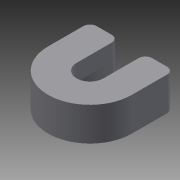
# Autodesk Inventor part: HeadConnector
Saved by Autodesk Inventor 2014 SP1 (Build 180222100, 222)
## iProperties
Created: 2013-10-30
Part Number: HeadConnector
Material: Generic
Document SubType Name: Modeling
Designer: david
Density: 1 g/cm^3
Appearance: Default
HeadConnectorDiam: 20,000 mm
HeadConnectorHeight: 5,000 mm
HeadConnectorOuterSize: 25,000 mm
HeadConnectorWidth: 8,000 mm
HeadConnectorOuterHeight: 5,000 mm
HeadConnectorTolerance: 0,200 mm
Author: david
Autodesk Inventor part; units mm, degrees
ref_plane "YZ Plane" through (0, 0, 0) normal (1, 0, 0) x (0, 1, 0)
ref_plane "XZ Plane" through (0, 0, 0) normal (0, 1, 0) x (-1, 0, 0)
ref_plane "XY Plane" through (0, 0, 0) normal (0, 0, 1) x (1, 0, 0)
sketch "Sketch1" plane through (0, 0, 0) normal (0, 1, 0) x (-1, 0, 0)
  arc A0 (12.5, 0) -> (-12.5, 0) centre (0, 0) ccw
  arc A1 (4, 0) -> (-4, 0) centre (0, 0) ccw
  line L0 (-12.5, 0) -> (12.5, 0) construction
  line L1 (0, 0) -> (0, -12.6122) construction
  line L2 (-12.5, 0) -> (-12.5, -12.5)
  line L3 (-4, 0) -> (-4, -12.5)
  line L4 (4, 0) -> (4, -12.5)
  line L5 (12.5, 0) -> (12.5, -12.5)
  line L6 (-12.5, -12.5) -> (-4, -12.5)
  line L7 (4, -12.5) -> (12.5, -12.5)
  dimension "d0" = 25
  dimension "d2" = 12.5
  dimension "d3" = 8
  dimension "d6" = 12.5
  dimension "d8" = 12.5
  constraints: 16 end point, 4 point on circle, 4 tangent, 3 parallel, 2 centre point, 2 coincident, 2 point on line, 1 horizontal, 1 perpendicular
  measures "d0" distance of L0.end L0.start
  measures "d2" radius of A0
  measures "d3" distance of L3.start L4.start
  measures "d6" distance of L2.end L0.start
  measures "d8" distance from line of L1.end L5
extrude "Extrusion1" add sketch "Sketch1" against normal blind 5
sketch "Sketch2" plane through (0, -5, 0) normal (0, -1, 0) x (1, 0, 0)
  arc A0 (12.5, 0) -> (-12.5, 0) centre (0, 0) ccw projected
  line L0 (-12.5, 0) -> (-12.5, -12.5) projected
  line L1 (-4, -12.5) -> (-4, 0) projected
  arc A1 (4, 0) -> (-4, 0) centre (0, 0) ccw projected
  line L2 (4, 0) -> (4, -12.5) projected
  line L3 (12.5, -12.5) -> (12.5, 0) projected
  arc A2 (4, -9.1652) -> (-4, -9.1652) centre (0, 0) ccw
  arc A3 (12.5, 0) -> (-12.5, 0) centre (0, 0) ccw
  line L4 (-12.5, 0) -> (-12.5, -12.5)
  line L5 (-4, -12.5) -> (-4, -9.1652)
  line L6 (4, -9.1652) -> (4, -12.5)
  line L7 (12.5, -12.5) -> (12.5, 0)
  line L8 (-12.5, -12.5) -> (-4, -12.5)
  line L9 (4, -12.5) -> (12.5, -12.5)
  dimension "d11" = 10
  constraints: 12 end point, 5 point on circle, 4 tangent, 3 collinear, 2 centre point, 2 coincident, 2 point on line, 1 parallel, 1 perpendicular
  measures "d11" radius of A2
extrude "Extrusion2" add sketch "Sketch2" along normal blind 5 contours L3 L9 L2 A2 L1 L8 L0 A0
fillet "Fillet1" radius 2 1 edges at (12.5, -5, -12.5)
fillet "Fillet2" radius 2 3 edges at (4, -5, -12.5) (-4, -5, -12.5) (-12.5, -5, -12.5)
sketch "Sketch3" plane through (0, -5, 0) normal (0, -1, 0) x (1, 0, 0)
  arc A0 (4, -9.1652) -> (-4, -9.1652) centre (0, 0) ccw projected
  line L0 (-4, -9.1652) -> (-4, 0) projected
  arc A1 (4, 0) -> (-4, 0) centre (0, 0) ccw projected
  line L1 (4, 0) -> (4, -9.1652) projected
  line L2 (0, 13.9059) -> (0, -15.9339) construction
  line L3 (-16.2747, -1.192) -> (17.4738, -7.1428) construction
  line L4 (-14.8856, 6.6864) -> (18.863, 0.7356) construction
  line L5 (-4, -19.239) -> (-4, 16.3727) construction
  line L6 (4, -9.1652) -> (4, -4.767)
  line L7 (8.3313, -5.5307) -> (4, -4.767)
  line L8 (-8.3313, 5.5307) -> (-4, 4.767)
  line L9 (-4, 9.1652) -> (-4, 4.767)
  arc A2 (-5, 8.6603) -> (-8.3313, 5.5307) centre (0, 0) ccw
  arc A3 (4, -9.1652) -> (8.3313, -5.5307) centre (0, 0) ccw
  dimension "d27" = 80
  constraints: 16 end point, 7 point on circle, 7 point on line, 3 collinear, 3 parallel, 2 centre point, 2 coincident, 2 tangent
  measures "d27" angle of L2 L4
extrude "Extrusion3" add sketch "Sketch3" along normal blind 5 contours L1 L7 A0 | L9 L8 A0
equation "\"d0\" = HeadConnectorOuterSize"
equation "\"d2\" = 0.5 * HeadConnectorOuterSize"
equation "\"d3\" = HeadConnectorWidth"
equation "\"d6\" = 0.5 * HeadConnectorOuterSize"
equation "\"d8\" = 0.5 * HeadConnectorOuterSize"
equation "\"d9\" = HeadConnectorOuterHeight"
equation "\"d11\" = 0.5 * HeadConnectorDiam"
equation "\"d12\" = HeadConnectorHeight"
equation "\"d28\" = HeadConnectorHeight"
equation "\"HeadConnectorDiam\" = 20"
equation "\"HeadConnectorWidth\" = 8"
equation "\"HeadConnectorOuterSize\" = 25"
equation "\"HeadConnectorHeight\" = 5"
equation "\"HeadConnectorOuterHeight\" = 5"
equation "\"HeadConnectorTolerance\" = 0.2"
body "Solid1"
